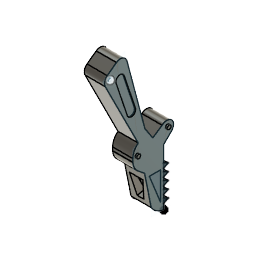
Jaw 7 (Gripper) (Autodesk Fusion 360 design; units mm, degrees)
part number: 2026-06-21-13-52-14-418
Autodesk Fusion 360 part; units mm, degrees
sketch "Sketch1" plane through (0, 0, 0) normal (1, 0, 0) x (0, 1, 0)
  line L0 (486.062, -71.899) -> (454.5004, -9.4181)
  line L1 (454.5004, -9.4181) -> (473.8363, 4.799)
  line L2 (473.8363, 4.799) -> (491.9855, -63.8421)
  line L3 (491.9855, -63.8421) -> (486.062, -71.899)
  line L4 (486.062, -71.899) -> (481.3021, -74.3713)
  line L5 (481.3021, -74.3713) -> (481.3021, -84.3713)
  line L6 (481.3021, -84.3713) -> (481.6163, -89.814)
  line L7 (497.6101, -127.3896) -> (497.6101, -134.3896)
  line L8 (497.6101, -134.3896) -> (508.6101, -134.3896)
  line L9 (508.6101, -134.3896) -> (508.6101, -84.3896)
  line L10 (508.6101, -84.3896) -> (515.6987, -77.3362)
  line L11 (481.6163, -89.814) -> (491.7399, -97.9696)
  line L12 (491.7399, -97.9696) -> (497.6101, -127.3896)
  line L13 (498.9415, -74.4178) -> (507.2345, -68.8298)
  line L14 (491.9855, -63.8421) -> (498.9415, -74.4178)
  arc A0 (515.6987, -77.3362) -> (507.2345, -68.8298) centre (511.4666, -73.083) ccw
  dimension "d1" = 70
  dimension "d2" = 24
  dimension "d3" = 71
  dimension "d4" = 15
  dimension "d5" = 10
  dimension "d6" = 10
  dimension "d7" = 13
  dimension "d8" = 30
  dimension "d9" = 7
  dimension "d10" = 11
  dimension "d11" = 10
  dimension "d12" = 50
  dimension "d14" = 10
  dimension "d15" = 12
  constraint vertical L5
  constraint parallel L5 L7
  constraint perpendicular L7 L8
  constraint perpendicular L8 L9
  constraint tangent L10 A0
  measures "d1" distance of L0.end L0.start
  measures "d2" distance of L0.end L1.end
  measures "d3" distance of L1.end L2.end
  measures "d4" distance of L2.end L4.end
  measures "d5" distance of L2.end L0.start
  measures "d6" distance of L4.end L5.end
  measures "d7" distance of L6.end L11.end
  measures "d8" distance of L7.start L11.end
  measures "d9" distance of L7.start L7.end
  measures "d10" distance of L7.end L8.end
  measures "d11" distance of L9.end L10.end
  measures "d12" distance of L8.end L9.end
  measures "d14" distance of L13.start L13.end
  measures "d15" distance of L10.end L13.end
extrude "Extrude1" add sketch "Sketch1" along normal mid plane 18
sketch "Sketch3" plane through (9, 0, 0) normal (1, 0, 0) x (0, 1, 0)
  line L0 (486.062, -71.899) -> (481.3021, -74.3713)
  line L1 (481.3021, -74.3713) -> (481.3021, -84.3713)
  line L2 (481.3021, -84.3713) -> (481.6163, -89.814)
  line L3 (481.6163, -89.814) -> (491.7399, -97.9696)
  line L4 (491.7399, -97.9696) -> (497.6101, -127.3896)
  line L5 (497.6101, -127.3896) -> (497.6101, -134.3896)
  line L6 (497.6101, -134.3896) -> (508.6101, -134.3896)
  line L7 (508.6101, -134.3896) -> (508.6101, -84.3896)
  line L8 (508.6101, -84.3896) -> (515.6987, -77.3362)
  arc A0 (515.6987, -77.3362) -> (507.2345, -68.8298) centre (511.4666, -73.083) ccw
  line L9 (507.2345, -68.8298) -> (498.9415, -74.4178)
  line L10 (498.9415, -74.4178) -> (491.9855, -63.8421)
  line L11 (491.9855, -63.8421) -> (473.8363, 4.799)
  line L12 (473.8363, 4.799) -> (454.5004, -9.4181)
  line L13 (454.5004, -9.4181) -> (486.062, -71.899)
  line L14 (497.6101, -127.3896) -> (505.9101, -127.3896)
  line L15 (505.9101, -127.3896) -> (505.9101, -102.3896)
  line L16 (505.9101, -102.3896) -> (495.9101, -102.3896)
  line L17 (495.9101, -102.3896) -> (505.9101, -127.3896)
  dimension "d18" = 25
  dimension "d19" = 10
  dimension "d20" = 2.7
  constraint coincident L4.end L5.start
  constraint perpendicular L5 L14
  constraint perpendicular L14 L15
  constraint perpendicular L15 L16
  measures "d18" distance of L14.end L15.end
  measures "d19" distance of L15.end L16.end
  measures "d20" distance of L7 L15
extrude "Extrude2" cut sketch "Sketch3" against normal blind 71 contours L15 L16 L17
sketch "Sketch4" plane through (9, 0, 0) normal (1, 0, 0) x (0, 1, 0)
  line L0 (505.9101, -102.3896) -> (505.9101, -127.3896)
  line L1 (505.9101, -127.3896) -> (495.9101, -102.3896)
  line L2 (495.9101, -102.3896) -> (505.9101, -102.3896)
  line L3 (486.062, -71.899) -> (481.3021, -74.3713)
  line L4 (481.3021, -74.3713) -> (481.3021, -84.3713)
  line L5 (481.3021, -84.3713) -> (481.6163, -89.814)
  line L6 (481.6163, -89.814) -> (491.7399, -97.9696)
  line L7 (491.7399, -97.9696) -> (497.6101, -127.3896)
  line L8 (497.6101, -127.3896) -> (497.6101, -134.3896)
  line L9 (497.6101, -134.3896) -> (508.6101, -134.3896)
  line L10 (508.6101, -134.3896) -> (508.6101, -84.3896)
  line L11 (508.6101, -84.3896) -> (515.6987, -77.3362)
  arc A0 (515.6987, -77.3362) -> (507.2345, -68.8298) centre (511.4666, -73.083) ccw
  line L12 (507.2345, -68.8298) -> (498.9415, -74.4178)
  line L13 (498.9415, -74.4178) -> (491.9855, -63.8421)
  line L14 (491.9855, -63.8421) -> (473.8363, 4.799)
  line L15 (473.8363, 4.799) -> (454.5004, -9.4181)
  line L16 (454.5004, -9.4181) -> (486.062, -71.899)
  line L17 (508.6101, -134.3896) -> (508.6101, -129.3896)
  line L18 (508.6101, -129.3896) -> (508.6101, -125.3896)
  line L19 (508.6101, -127.3896) -> (512.6101, -127.3896)
  line L20 (508.6101, -125.3896) -> (512.6101, -127.3896)
  line L21 (512.6101, -127.3896) -> (508.6101, -129.3896)
  line L22 (508.6101, -118.6396) -> (512.6101, -120.6396)
  line L23 (512.6101, -120.6396) -> (508.6101, -122.6396)
  line L24 (508.6101, -122.6396) -> (508.6101, -118.6396)
  line L25 (508.6101, -111.8896) -> (512.6101, -113.8896)
  line L26 (512.6101, -113.8896) -> (508.6101, -115.8896)
  line L27 (508.6101, -115.8896) -> (508.6101, -111.8896)
  line L28 (508.6101, -105.1396) -> (512.6101, -107.1396)
  line L29 (512.6101, -107.1396) -> (508.6101, -109.1396)
  line L30 (508.6101, -109.1396) -> (508.6101, -105.1396)
  line L31 (508.6101, -98.3896) -> (512.6101, -100.3896)
  line L32 (512.6101, -100.3896) -> (508.6101, -102.3896)
  line L33 (508.6101, -102.3896) -> (508.6101, -98.3896)
  dimension "d23" = 5
  dimension "d24" = 4
  dimension "d25" = 4
  dimension "d30" = 0
  dimension "d31" = 27
  constraint coincident L9.end L10.start
  constraint perpendicular L9 L17
  constraint parallel L10 L18
  constraint midpoint L18 L19.start
  constraint perpendicular L18 L19
  measures "d23" distance of L9.end L17.end
  measures "d24" distance of L17.end L18.end
  measures "d25" distance of L19.start L19.end
extrude "Extrude3" add sketch "Sketch4" against normal up to surface (18 mm away) contours L10 L18 L19 L21 | L10 L18 L19 L20
extrude "Extrude4" add sketch "Sketch4" against normal up to surface (18 mm away) contours L10 L31 L32 L33 | L10 L28 L29 L30 | L10 L22 L23 L24 | L10 L25 L26 L27
fillet "Fillet1" radius 6 2 edges at (0, 473.8363, 4.799) (0, 454.5004, -9.4181)
fillet "Fillet2" radius 15 1 edges at (0, 497.6101, -134.3896)
fillet "Fillet3" radius 12 2 edges at (0, 481.3021, -74.3713) (0, 481.6163, -89.814)
sketch "Sketch5" plane through (9, 0, 0) normal (1, 0, 0) x (0, 1, 0)
  arc A0 (481.3095, -84.5001) -> (485.7614, -93.1532) centre (493.2896, -83.8084) ccw
  line L0 (485.7614, -93.1532) -> (491.7399, -97.9696)
  line L1 (491.7399, -97.9696) -> (497.6101, -127.3896)
  arc A1 (497.6101, -127.3896) -> (508.6101, -134.3896) centre (510.3629, -119.4924) ccw
  line L2 (508.6101, -134.3896) -> (508.6101, -129.3896)
  line L3 (508.6101, -129.3896) -> (512.6101, -127.3896)
  line L4 (512.6101, -127.3896) -> (508.6101, -125.3896)
  line L5 (508.6101, -125.3896) -> (508.6101, -122.6396)
  line L6 (508.6101, -122.6396) -> (512.6101, -120.6396)
  line L7 (512.6101, -120.6396) -> (508.6101, -118.6396)
  line L8 (508.6101, -118.6396) -> (508.6101, -115.8896)
  line L9 (508.6101, -115.8896) -> (512.6101, -113.8896)
  line L10 (512.6101, -113.8896) -> (508.6101, -111.8896)
  line L11 (508.6101, -111.8896) -> (508.6101, -109.1396)
  line L12 (508.6101, -109.1396) -> (512.6101, -107.1396)
  line L13 (512.6101, -107.1396) -> (508.6101, -105.1396)
  line L14 (508.6101, -105.1396) -> (508.6101, -102.3896)
  line L15 (508.6101, -102.3896) -> (512.6101, -100.3896)
  line L16 (512.6101, -100.3896) -> (508.6101, -98.3896)
  line L17 (508.6101, -98.3896) -> (508.6101, -84.3896)
  line L18 (508.6101, -84.3896) -> (515.6987, -77.3362)
  arc A2 (515.6987, -77.3362) -> (507.2345, -68.8298) centre (511.4666, -73.083) ccw
  line L19 (507.2345, -68.8298) -> (498.9415, -74.4178)
  line L20 (498.9415, -74.4178) -> (491.9855, -63.8421)
  line L21 (491.9855, -63.8421) -> (476.0895, -3.7229)
  arc A3 (476.0895, -3.7229) -> (466.7346, -0.4226) centre (470.2889, -5.2566) ccw
  line L22 (466.7346, -0.4226) -> (458.5908, -6.4105)
  arc A4 (458.5908, -6.4105) -> (456.7896, -13.9498) centre (462.1451, -11.2445) ccw
  line L23 (456.7896, -13.9498) -> (486.062, -71.899)
  arc A5 (486.062, -71.899) -> (481.3021, -81.4688) centre (493.3021, -81.4688) ccw
  line L24 (481.3021, -81.4688) -> (481.3021, -84.3713)
  line L25 (481.3021, -84.3713) -> (481.3095, -84.5001)
  line L26 (505.9101, -102.3896) -> (505.9101, -127.3896)
  line L27 (505.9101, -127.3896) -> (495.9101, -102.3896)
  line L28 (495.9101, -102.3896) -> (505.9101, -102.3896)
  circle A6 centre (461, -11) radius 1.5
  dimension "d40" = 3
  measures "d40" diameter of A6
extrude "Extrude5" cut sketch "Sketch5" against normal blind 33 contours A6
sketch "Sketch7" plane through (0, 454.1129, 90.609) normal (0, -0.980669, -0.195673) x (1, 0, 0)
  line L0 (-9, -222.2957) -> (9, -222.2957)
  line L1 (9, -222.2957) -> (9, -192.2957)
  line L2 (9, -192.2957) -> (-9, -192.2957)
  line L3 (-9, -192.2957) -> (-9, -222.2957)
  line L4 (-6, -199.7367) -> (6, -199.7367)
  line L5 (6, -199.7367) -> (9, -199.7367)
  line L6 (-6, -199.7367) -> (-9, -199.7367)
  line L7 (3.1939, -218.0429) -> (-2.6041, -218.0429)
  line L8 (-6, -199.7367) -> (-2.6041, -218.0429)
  line L9 (6, -199.7367) -> (3.1939, -218.0429)
  dimension "d43" = 3
  dimension "d44" = 3
  dimension "d45" = 7.441
  constraint parallel L0 L4
  constraint coincident L1 L5.end
  constraint perpendicular L1 L5
  constraint coincident L3 L6.end
  constraint perpendicular L3 L6
  constraint parallel L4 L7
  measures "d43" distance of L4.start L6.end
  measures "d44" distance of L4.end L5.end
  measures "d45" distance of L2 L4
extrude "Extrude6" cut sketch "Sketch7" against normal blind 9 contours L4 L7 L8 L9
sketch "Sketch8" plane through (9, 0, 0) normal (1, 0, 0) x (0, 1, 0)
  circle A0 centre (512, -72) radius 1.75
  circle A1 centre (485, -81) radius 1.75
  dimension "d48" = 3.5
  dimension "d49" = 3.5
  measures "d48" diameter of A0
  measures "d49" diameter of A1
extrude "Extrude7" add sketch "Sketch8" along normal blind 1.5
sketch "Sketch9" plane through (9, 0, 0) normal (1, 0, 0) x (0, 1, 0)
  line L0 (466.432, -16.1893) -> (476.432, -46.1893)
  arc A0 (476.432, -46.1893) -> (483.568, -43.8107) centre (480, -45) ccw
  line L1 (483.568, -43.8107) -> (473.568, -13.8107)
  arc A1 (473.568, -13.8107) -> (466.432, -16.1893) centre (470, -15) ccw
  line L2 (470, -15) -> (480, -45) construction
  dimension "d52" = 7.522
  constraint tangent L0 A0
  constraint tangent A0 L1
  constraint parallel L0 L1
  constraint tangent L1 A1
  constraint tangent L0 A1
  measures "d52" diameter of A0
extrude "Extrude8" cut sketch "Sketch9" against normal blind 1
ref_plane "WorkPlane1" through (0, 487.2262, -64.7953) normal (-1, 0, 0) x (0, -1, 0)
mirror "Mirror1" about plane through (0, 487.2262, -64.7953) normal (-1, 0, 0) of "Extrude7", "Extrude8"
